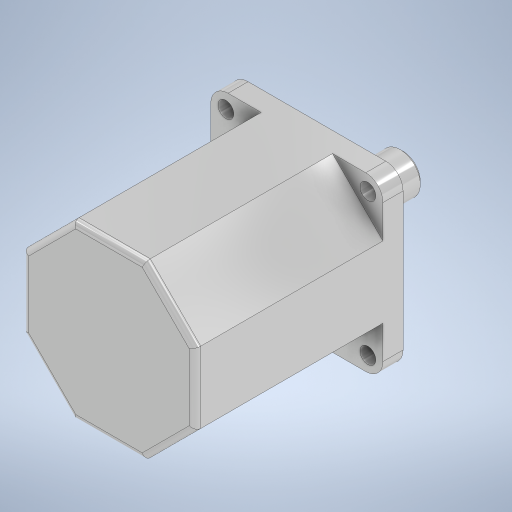
# Autodesk Inventor part: silnik_podstawa
Saved by Autodesk Inventor 2023 (Build 270158000, 158)
## iProperties
Created: 2023-03-29
Part Number: silnik_podstawa
Material: Aluminium 6061-AHC
Document SubType Name: Modeling
Designer: krzys
Density: 2.7 g/cm^3
Appearance: Aluminium — ciemne
Author: krzys
Autodesk Inventor part; units mm, degrees
ref_plane "YZ Plane" through (0, 0, 0) normal (1, 0, 0) x (0, 1, 0)
ref_plane "XZ Plane" through (0, 0, 0) normal (0, 1, 0) x (-1, 0, 0)
ref_plane "XY Plane" through (0, 0, 0) normal (0, 0, 1) x (1, 0, 0)
sketch "Szkic1" plane through (0, 0, 0) normal (0, 0, 1) x (1, 0, 0)
  circle A0 centre (0, 0) radius 25
  circle A1 centre (0, 0) radius 7
  line L0 (-24, 30) -> (24, 30)
  line L1 (30, 24) -> (30, -24)
  line L2 (24, -30) -> (-24, -30)
  line L3 (-30, -24) -> (-30, 24)
  line L4 (-30, 30) -> (30, -30) construction
  line L5 (30, 30) -> (-30, -30) construction
  circle A2 centre (-24.7487, 24.7487) radius 2.75
  circle A3 centre (24.7487, 24.7487) radius 2.75
  circle A4 centre (-24.7487, -24.7487) radius 2.75
  circle A5 centre (24.7487, -24.7487) radius 2.75
  arc A6 (-24, 30) -> (-30, 24) centre (-24, 24) ccw
  arc A7 (30, 24) -> (24, 30) centre (24, 24) ccw
  arc A8 (24, -30) -> (30, -24) centre (24, -24) ccw
  arc A9 (-30, -24) -> (-24, -30) centre (-24, -24) ccw
  dimension "d0" = 50
  dimension "d1" = 14
  dimension "d2" = 60
  dimension "d3" = 60
  dimension "d5" = 5.5
  dimension "d6" = 5.5
  dimension "d7" = 5.5
  dimension "d8" = 5.5
  dimension "d9" = 6
  constraints: 12 end point, 10 centre point, 8 point on circle, 8 point on line, 8 tangent, 3 equal radius, 2 coincident, 2 midpoint, 2 parallel, 1 horizontal, 1 perpendicular
  measures "d0" diameter of A0
  measures "d1" diameter of A1
  measures "d2" distance of L4.end L5.end
  measures "d3" distance of L5.start L4.end
  measures "d5" diameter of A2
  measures "d6" diameter of A3
  measures "d7" diameter of A4
  measures "d8" diameter of A5
  measures "d9" radius of A6
extrude "Wyciągnięcie proste1" add sketch "Szkic1" along normal blind 7 contours A0 | A1 | L0 A7 L1 A8 L2 A9 L3 A6
extrude "Wyciągnięcie proste2" add sketch "Szkic1" against normal blind 3 contours A0
extrude "Wyciągnięcie proste3" add sketch "Szkic1" against normal blind 30 contours A1
sketch "Szkic2" plane through (0, 0, 7) normal (0, 0, 1) x (1, 0, 0)
  line L0 (-30, 12.4264) -> (-12.4264, 30)
  line L1 (12.4264, 30) -> (30, 12.4264)
  line L2 (30, -12.4264) -> (12.4264, -30)
  line L3 (-12.4264, -30) -> (-30, -12.4264)
  line L4 (-30, 30) -> (30, -30) construction
  line L5 (30, 30) -> (-30, -30) construction
  line L6 (-12.4264, 30) -> (12.4264, 30)
  line L7 (30, -24) -> (30, 24) projected
  line L8 (30, 12.4264) -> (30, -12.4264)
  line L9 (-24, -30) -> (24, -30) projected
  line L10 (12.4264, -30) -> (-12.4264, -30)
  line L11 (-30, 24) -> (-30, -24) projected
  line L12 (-30, -12.4264) -> (-30, 12.4264)
  point P0 (0, 0)
  constraints: 20 end point, 6 point on line, 2 midpoint, 2 parallel, 1 horizontal, 1 perpendicular
extrude "Wyciągnięcie proste4" add sketch "Szkic2" along normal blind 65.5
fillet "Zaokrąglenie1" radius 2 8 edges at (30, 0, 72.5) (21.2132, 21.2132, 72.5) (0, 30, 72.5) (-21.2132, 21.2132, 72.5) (-30, 0, 72.5) (21.2132, -21.2132, 72.5) (0, -30, 72.5) (-21.2132, -21.2132, 72.5)
chamfer "Faza1" distance 1 angle 45 1 edges at (-7, 0, -30)
